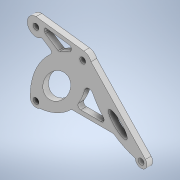
# Autodesk Inventor part: Bracket Design MK29
Saved by Autodesk Inventor 2021 (Build 250183000, 183)
## iProperties
Created: 2021-05-08
Part Number: Bracket Design MK29
Material: Generic
Document SubType Name: Modeling
Designer: Nabeel Azafer
Density: 1 g/cm^3
Appearance: Default
Author: Nabeel Azafer
Autodesk Inventor part; units mm, degrees
ref_plane "YZ Plane" through (0, 0, 0) normal (1, 0, 0) x (0, 1, 0)
ref_plane "XZ Plane" through (0, 0, 0) normal (0, 1, 0) x (-1, 0, 0)
ref_plane "XY Plane" through (0, 0, 0) normal (0, 0, 1) x (1, 0, 0)
sketch "Sketch1" plane through (0, 0, 0) normal (0, 0, 1) x (1, 0, 0)
  line L0 (-110, 75) -> (110, 75)
  line L1 (110, 75) -> (110, -75)
  line L2 (110, -75) -> (-110, -75)
  line L3 (-110, -75) -> (-110, 75)
  circle A0 centre (-90, 55) radius 5
  circle A1 centre (-90, -55) radius 5
  circle A2 centre (-10, 45) radius 5
  circle A3 centre (90, -55) radius 5
  line L4 (-67, 0) -> (-42, 0)
  line L5 (-42, 0) -> (-42, -30) construction
  line L6 (-42, -30) -> (-67, -30) construction
  line L7 (-67, -30) -> (-67, 0) construction
  line L8 (40, -10) -> (60, -10) construction
  line L9 (60, -10) -> (60, -30) construction
  line L10 (60, -30) -> (40, -30) construction
  line L11 (40, -30) -> (40, -10) construction
  arc A4 (80, -55) -> (97.2566, -48.1194) centre (90, -55) ccw
  line L12 (-78.6576, 42.7238) -> (-65.8852, 34.4414)
  line L13 (-73.8616, 52.6815) -> (-52.1474, 38.6008)
  arc A5 (-32.4903, 47.1034) -> (-49.4708, 38.573) centre (6.8085, -52.2903) ccw
  arc A6 (-65.2329, 26.555) -> (-99.9598, -54.9486) centre (6.8085, -52.2903) ccw
  arc A7 (4.0877, 50.1405) -> (-8.1602, 59.8829) centre (-10, 45) ccw
  arc A8 (-99.9598, -54.9486) -> (-84.0979, -63.0229) centre (-90, -55) ccw
  arc A9 (-65.2329, 26.555) -> (-65.8852, 34.4414) centre (-68.6056, 30.2462) ccw
  arc A10 (-78.6576, 42.7238) -> (-81.4438, 42.6796) centre (-80.0178, 40.6262) ccw
  arc A11 (-75.0012, 54.8107) -> (-73.8616, 52.6815) centre (-72.5014, 54.7791) ccw
  arc A12 (-52.1474, 38.6008) -> (-49.4708, 38.573) centre (-50.7872, 40.6984) ccw
  line L14 (4.0877, 50.1405) -> (97.2566, -48.1194)
  line L15 (-90, 70) -> (-8.1602, 59.8829)
  line L16 (-72.6683, 61.5308) -> (-33.7153, 56.7154)
  arc A13 (-72.6683, 61.5308) -> (-75.4072, 58.4711) centre (-72.975, 59.0497) ccw
  arc A14 (-32.4903, 47.1034) -> (-33.7153, 56.7154) centre (-34.3288, 51.7532) ccw
  arc A15 (-75.0012, 54.8107) -> (-75.4072, 58.4711) centre (-90, 55) ccw
  arc A16 (-86.3472, 69.5484) -> (-81.4438, 42.6796) centre (-90, 55) ccw
  arc A17 (7.2449, 4.5703) -> (-6.7415, 3.0356) centre (0.5352, 1.2191) ccw
  circle A18 centre (-54.5, -15) radius 10 construction
  ellipse E0 centre (-54.5, -15) end of major axis (-34.8909, 8.7663) minor radius 17.7603
  ellipse E1 centre (50, -20) end of major axis (34.7246, -5) minor radius 7.7204
  circle A19 centre (43.0635, -13.1154) radius 3 construction
  circle A20 centre (47.4663, -17.5409) radius 3 construction
  circle A21 centre (51.9204, -22.0998) radius 3 construction
  circle A22 centre (56.7938, -26.2396) radius 3 construction
  line L17 (-13.3698, -30) -> (21.5888, -30)
  line L18 (-29.4124, -37.1956) -> (42.7303, -37.1956)
  arc A23 (-84.0979, -63.0229) -> (-29.4124, -37.1956) centre (-92.0008, 24.5184) ccw
  arc A24 (-17.6007, -22.3356) -> (-6.7415, 3.0356) centre (-92.0008, 24.5184) ccw
  arc A25 (7.2449, 4.5703) -> (25.2764, -21.6234) centre (110.2095, 56.1472) ccw
  arc A26 (42.7303, -37.1956) -> (80, -55) centre (110.2095, 56.1472) ccw
  arc A27 (-17.6007, -22.3356) -> (-13.3698, -30) centre (-13.3698, -25) ccw
  arc A28 (21.5888, -30) -> (25.2764, -21.6234) centre (21.5888, -25) ccw
  point P0 (0, 0)
  dimension "d0" = 220
  dimension "d1" = 150
  dimension "d6" = 10
  dimension "d8" = 55
  dimension "d9" = 10
  dimension "d10" = 10
  dimension "d11" = 10
  dimension "d15" = 90
  dimension "d16" = 90
  dimension "d17" = 55
  dimension "d19" = 75
  dimension "d21" = 0
  dimension "d26" = 20
  dimension "d27" = 10
  dimension "d30" = 55
  dimension "d95" = 10
  dimension "d96" = 45
  dimension "d97" = 90
  dimension "d100" = 20
  dimension "d101" = 42
  dimension "d102" = 30
  dimension "d103" = 25
  dimension "d104" = 20
  dimension "d105" = 50
  dimension "d106" = 40
  dimension "d112" = 10
  dimension "d113" = 5
  dimension "d114" = 5
  dimension "d115" = 5
  dimension "d125" = 5
  dimension "d126" = 10
  dimension "d131" = 15
  dimension "d132" = 20
  dimension "d133" = 6
  dimension "d134" = 6
  dimension "d135" = 6
  dimension "d136" = 6
  dimension "d139" = 10
  dimension "d140" = 10
  constraints: 41 point on circle, 38 end point, 30 centre point, 15 tangent, 9 parallel, 5 coincident, 4 perpendicular, 3 horizontal, 1 point on line, 2 other
  measures "d0" distance of L1.end L2.end
  measures "d1" distance of L2.end L0.start
  measures "d6" diameter of A0
  measures "d8" vertical distance of point (0, 0) A1.centre
  measures "d9" diameter of A1
  measures "d10" diameter of A3
  measures "d11" diameter of A2
  measures "d15" horizontal distance of point (0, 0) A3.centre
  measures "d16" horizontal distance of point (0, 0) A1.centre
  measures "d17" vertical distance of A0.centre point (0, 0)
  measures "d19" distance from line of point (0, 0) L0
  measures "d21" distance from line of point (0, 0) L4
  measures "d26" distance of L8.end L9.end
  measures "d27" distance from line of point (0, 0) L8
  measures "d30" vertical distance of point (0, 0) A3.centre
  measures "d95" horizontal distance of point (0, 0) A2.centre
  measures "d96" vertical distance of point (0, 0) A2.centre
  measures "d97" horizontal distance of point (0, 0) A0.centre
  measures "d100" diameter of A4
  measures "d101" distance from line of point (0, 0) L5
  measures "d102" distance of L6.end L4.start
  measures "d103" distance of L4.start L4.end
  measures "d104" distance of L9.end L10.end
  measures "d105" distance between parallel lines of L1 L9
  measures "d106" distance from line of point (0, 0) L11
  measures "d112" diameter of A9
  measures "d113" diameter of A10
  measures "d114" diameter of A11
  measures "d115" diameter of A12
  measures "d125" diameter of A13
  measures "d126" diameter of A14
  measures "d131" diameter of A17
  measures "d132" diameter of A18
  measures "d133" diameter of A19
  measures "d134" diameter of A20
  measures "d135" diameter of A21
  measures "d136" diameter of A22
  measures "d139" diameter of A27
  measures "d140" diameter of A28
extrude "Extrusion22" add sketch "Sketch1" along normal blind 9.725 contours A26 L18 A23 A8 A6 A9 L12 A10 A16 L15 A7 L14 A4
body "Solid21"
